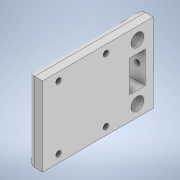
# Autodesk Inventor part: Joint_Tubes_1_3
Saved by Autodesk Inventor 2022.3 (Build 263350000, 350)
## iProperties
Created: 2023-05-15
Part Number: Joint_Tubes_1_3
Material: Generic
Document SubType Name: Modeling
Designer: Manuel Hueso Béjar
Density: 1 g/cm^3
Appearance: Default
Author: Manuel Hueso Béjar
Autodesk Inventor part; units mm, degrees
ref_plane "YZ Plane" through (0, 0, 0) normal (1, 0, 0) x (0, 1, 0)
ref_plane "XZ Plane" through (0, 0, 0) normal (0, 1, 0) x (-1, 0, 0)
ref_plane "XY Plane" through (0, 0, 0) normal (0, 0, 1) x (1, 0, 0)
sketch "Sketch1" plane through (0, 0, 0) normal (0, 1, 0) x (-1, 0, 0)
  line L0 (-5, 35) -> (5, 35)
  line L1 (5, 35) -> (5, -35)
  line L2 (5, -35) -> (-5, -35)
  line L3 (-5, -35) -> (-5, 35)
  line L4 (-5, 35) -> (5, -35) construction
  line L5 (5, 35) -> (-5, -35) construction
  point P0 (0, 0)
  dimension "d0" = 10
  dimension "d1" = 70
  constraints: 12 end point, 2 midpoint, 2 parallel, 1 horizontal, 1 perpendicular
  measures "d0" distance of L1.end L2.end
  measures "d1" distance of L0.end L1.end
extrude "Extrusion1" add sketch "Sketch1" along normal blind 50
sketch "Sketch2" plane through (-5, 0, -35) normal (-1, 0, 0) x (0, 0, 1)
  line L0 (0, 0) -> (70, 0) projected
  line L1 (0, 50) -> (20, 50)
  line L2 (20, 50) -> (20, 0)
  line L3 (20, 0) -> (0, 0)
  line L4 (0, 0) -> (0, 50)
  line L5 (0, 50) -> (70, 50) projected
  line L6 (10, 50) -> (10, 42.5)
  line L7 (10, 0) -> (10, 7.5)
  line L8 (10, 0) -> (17.5, 0) construction
  circle A0 centre (10, 42.5) radius 4.1
  circle A1 centre (10, 42.5) radius 6
  circle A2 centre (10, 7.5) radius 4.1
  circle A3 centre (10, 7.5) radius 6
  line L9 (70, 0) -> (0, 0) projected
  line L10 (5, 15) -> (15, 15)
  line L11 (15, 15) -> (15, 35)
  line L12 (15, 35) -> (5, 35)
  line L13 (5, 35) -> (5, 15)
  line L14 (5, 15) -> (15, 35) construction
  line L15 (15, 15) -> (5, 35) construction
  point P0 (35, 0)
  point P1 (10, 25)
  dimension "d4" = 20
  dimension "d5" = 7.5
  dimension "d6" = 7.5
  dimension "d7" = 90
  dimension "d8" = 8.2
  dimension "d9" = 12
  dimension "d10" = 8.2
  dimension "d11" = 12
  dimension "d12" = 10
  dimension "d13" = 20
  constraints: 26 end point, 4 centre point, 4 coincident, 4 parallel, 4 perpendicular, 3 horizontal, 3 midpoint, 2 point on line, 1 vertical
  measures "d4" distance of L2.end L3.end
  measures "d5" distance of L6.start L6.end
  measures "d6" distance of L7.start L7.end
  measures "d7" angle of L8 L7
  measures "d8" diameter of A0
  measures "d9" diameter of A1
  measures "d10" diameter of A2
  measures "d11" diameter of A3
  measures "d12" distance of L12.end L11.end
  measures "d13" distance of L11.end L10.end
extrude "Extrusion2" cut sketch "Sketch2" against normal through all contours A0 | A2 | L13 L12 L11 L10
extrude "Extrusion3" cut sketch "Sketch2" against normal blind 2 contours A1 | A3
sketch "Sketch3" plane through (-5, 0, -35) normal (-1, 0, 0) x (0, 0, 1)
  line L0 (70, 0) -> (70, 50) projected
  line L1 (70, 50) -> (60, 50)
  line L2 (60, 50) -> (60, 45)
  line L3 (60, 45) -> (70, 45)
  line L4 (70, 45) -> (70, 50)
  line L5 (60, 45) -> (30, 45)
  line L6 (30, 45) -> (30, 5)
  line L7 (30, 5) -> (60, 5)
  line L8 (60, 5) -> (60, 45)
  point P0 (35, 0)
  dimension "d18" = 10
  dimension "d19" = 5
  dimension "d20" = 30
  dimension "d21" = 40
  constraints: 16 end point, 4 parallel, 2 horizontal, 2 perpendicular
  measures "d18" distance of L3.end L2.end
  measures "d19" distance of L2.end L1.end
  measures "d20" distance of L7.end L6.end
  measures "d21" distance of L6.end L5.end
hole "Hole1" at (-5, 45, 25) at (-5, 45, -5) at (-5, 5, -5) at (-5, 5, 25) direction (1, 0, 0) diameter 3.4 end through all countersink diameter 5.9 countersink angle 90
sketch "Sketch4" plane through (5, 0, -35) normal (0, 0, -1) x (-1, 0, 0)
  line L0 (0, 15) -> (0, 35) projected
  line L1 (0, 0) -> (0, 50) projected
  line L2 (0, 25) -> (10, 25)
  line L3 (10, 0) -> (10, 50) projected
  line L4 (5, 25) -> (5, 20)
  line L5 (5, 25) -> (10, 25) construction
  point P0 (5, 0)
  dimension "d30" = 5
  dimension "d31" = 90
  constraints: 6 end point, 3 midpoint, 1 horizontal, 1 perpendicular, 1 vertical
  measures "d30" distance of L4.start L4.end
  measures "d31" angle of L4 L5
fillet "Fillet1" radius 5 4 edges at (-5, 50, 0) (-5, 25, -35) (-5, 0, 0) (-5, 25, 35)
hole "Hole2" at (0, 25, -35) direction (0, 0, 1) diameter 3.4 depth 5 countersink diameter 5.9 countersink angle 90
sketch "Sketch5" plane through (-5, 15, -20) normal (0, 0, -1) x (-1, 0, 0)
  line L0 (-10, 0) -> (-10, 20) projected
  line L1 (0, 20) -> (-10, 20) projected
  line L2 (-10, 0) -> (0, 20)
  line L3 (-5, 10) -> (-10, 10)
  point P0 (-5, -15)
  constraints: 4 end point, 2 midpoint
hole "Hole3" at (0, 25, -20) direction (0, 0, 1) diameter 3.4 depth 12 counterbore diameter 4.1 counterbore depth 5.1
body "Solid1"
